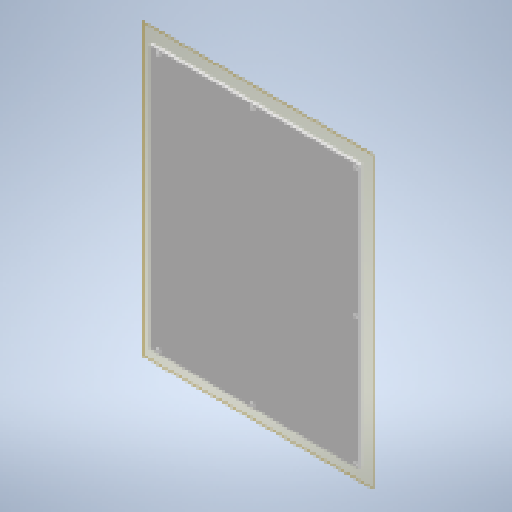
# Autodesk Inventor part: controller-top
Saved by Autodesk Inventor 2025.2 (Build 292293000, 293)
## iProperties
Created: 2025-04-21
Part Number: controller-top
Material: Generic
Document SubType Name: Modeling
Designer: tdeboutte
Density: 1 g/cm^3
Appearance: Default
Author: tdeboutte
Autodesk Inventor part; units mm, degrees
ref_plane "YZ Plane" through (0, 0, 0) normal (1, 0, 0) x (0, 1, 0)
ref_plane "XZ Plane" through (0, 0, 0) normal (0, 1, 0) x (-1, 0, 0)
ref_plane "XY Plane" through (0, 0, 0) normal (0, 0, 1) x (1, 0, 0)
ref_plane "Work Plane1" through (0, 0, 0) normal (0, 0, 1) x (1, 0, 0)
sketch "Sketch1" plane through (0, 0, 0) normal (0, 0, 1) x (1, 0, 0)
  circle A0 centre (-1, 73.25) radius 1.05 projected
  circle A1 centre (-54.8, -73.25) radius 1.05 projected
  circle A2 centre (-54.8, 73.25) radius 1.05 projected
  circle A3 centre (-1, -73.25) radius 1.05 projected
  circle A4 centre (58, -73.25) radius 1.05 projected
  circle A5 centre (58, 0) radius 1.05 projected
  circle A6 centre (58, 73.25) radius 1.05 projected
  line L0 (-60, -75.25) -> (60, -75.25) projected
  line L1 (60, -75.25) -> (60, 75.25) projected
  line L2 (60, 75.25) -> (-60, 75.25) projected
  line L3 (-60, 75.25) -> (-60, 73.25) projected
  line L4 (-60, 73.25) -> (-56.8, 73.25) projected
  line L5 (-56.8, 71.25) -> (-56.8, 73.25) projected
  line L6 (-54.8, 71.25) -> (-56.8, 71.25) projected
  arc A7 (-54.8, 71.25) -> (-52.8, 73.25) centre (-54.8, 73.25) ccw projected
  line L7 (-52.8, 73.25) -> (-3, 73.25) projected
  arc A8 (-3, 73.25) -> (1, 73.25) centre (-1, 73.25) ccw projected
  line L8 (1, 73.25) -> (56, 73.25) projected
  arc A9 (56, 73.25) -> (58, 71.25) centre (58, 73.25) ccw projected
  line L9 (58, 71.25) -> (58, 2) projected
  arc A10 (58, 2) -> (58, -2) centre (58, 0) ccw projected
  line L10 (58, -2) -> (58, -71.25) projected
  arc A11 (58, -71.25) -> (56, -73.25) centre (58, -73.25) ccw projected
  line L11 (56, -73.25) -> (1, -73.25) projected
  arc A12 (1, -73.25) -> (-3, -73.25) centre (-1, -73.25) ccw projected
  line L12 (-3, -73.25) -> (-52.8, -73.25) projected
  arc A13 (-52.8, -73.25) -> (-54.8, -71.25) centre (-54.8, -73.25) ccw projected
  line L13 (-56.8, -71.25) -> (-54.8, -71.25) projected
  line L14 (-56.8, -73.25) -> (-56.8, -71.25) projected
  line L15 (-56.8, -73.25) -> (-60, -73.25) projected
  line L16 (-60, -73.25) -> (-60, -75.25) projected
  line L17 (-56.8, -73.25) -> (-56.8, 73.25) projected
  line L18 (-56.8, 73.25) -> (-59.8, 73.25) projected
  line L19 (-59.8, -73.25) -> (-59.8, 73.25) projected
  line L20 (-56.8, -73.25) -> (-59.8, -73.25) projected
  line L21 (60, 75.25) -> (-60, 75.25)
  line L22 (-60, 75.25) -> (-60, -75.25)
  line L23 (-60, -75.25) -> (60, -75.25)
  line L24 (60, -75.25) -> (60, 75.25)
  point P0 (0, 0)
  constraints: 8 end point, 2 parallel, 1 horizontal, 1 perpendicular
extrude "Extrusion1" add sketch "Sketch1" along normal blind 2 contours A0 | A1 | A2 | A3 | A4 | A5 | A6 | L16 L15 L14 L13 A13 L12 A12 L11 A11 L10 A10 L9 A9 L8 A8 L7 A7 L6 L5 L4 L3 L2 L1 L0 | L22 L4 L19 L15 | L19 L4 L5 L17 L14 L15 | L17 L6 A7 L7 A8 L8 A9 L9 A10 L10 A11 L11 A12 L12 A13 L13
hole "Hole1" at (58, 73.25, 2) at (58, 0, 2) at (58, -73.25, 2) at (-1, -73.25, 2) at (-54.8, -73.25, 2) at (-54.8, 73.25, 2) at (-1, 73.25, 2) direction (0, 0, -1) diameter 2.2 depth 2
body "Solid1"
